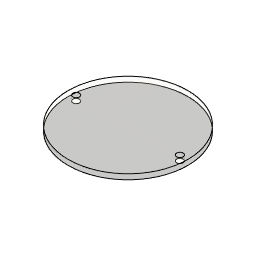
UNIT, SENSOR (L) (Autodesk Fusion 360 archive; units mm, degrees)
design "PLATE, COVER"
Autodesk Fusion 360 part; units mm, degrees
note: some values were not read from the file. Chosen so that the rebuilt part matches the saved one: which sketch regions a step uses.
sketch "Sketch1" plane through (0, 0, 0) normal (0, 1, 0) x (1, 0, 0)
  circle A0 centre (0, 0) radius 34.55
  dimension "d1" = 69.1
  constraint coincident A0.centre origin
  measures "d1" diameter of A0
extrude "Extrude1" add sketch "Sketch1" along normal blind 3
sketch "Sketch2" plane through (0, 3, 0) normal (0, 1, 0) x (-1, 0, 0)
  circle A0 centre (0, 0) radius 34.55
  line L0 (30, 0) -> (-30, 0) construction
  dimension "d4" = 60
  constraint horizontal L0
  constraint midpoint A0.centre L0
  measures "d4" distance of L0.start L0.end
hole "Hole1" at (-30, 3, 0) at (30, 3, 0) direction (0, -1, 0) diameter 3.8 end through all

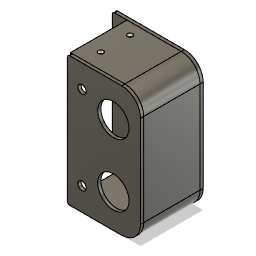
design "COVER, FIXTURE"
Autodesk Fusion 360 part; units mm, degrees
sketch "Sketch1" plane through (0, 0, 0) normal (0, 0, 1) x (1, 0, 0)
  line L0 (0, 31) -> (0, -31)
  line L1 (0, 31) -> (42, 31)
  line L2 (0, -31) -> (42, -31)
  line L3 (42, 31) -> (42, -31)
  dimension "d1" = 62
  dimension "d2" = 42
  constraint vertical L0
  constraint midpoint origin L0
  constraint perpendicular L0 L1
  constraint perpendicular L0 L2
  constraint perpendicular L1 L3
  measures "d1" distance of L0.start L0.end
  measures "d2" distance of L0.end L2.end
extrude "Extrude1" add sketch "Sketch1" along normal blind 1.5 makes body 1
fillet "Fillet3" radius 9 2 edges at (42, 31, 0.75) (42, -31, 0.75) on bodies 1
sketch "Sketch3" plane through (0, 0, 1.5) normal (0, 0, 1) x (1, 0, 0)
  arc A0 (33, -31) -> (42, -22) centre (33, -22) ccw
  line L0 (42, -22) -> (42, 22)
  arc A1 (42, 22) -> (33, 31) centre (33, 22) ccw
  line L1 (33, 31) -> (0, 31)
  line L2 (0, 31) -> (0, -31)
  line L3 (0, -31) -> (33, -31)
  line L4 (1.5, -29.5) -> (33, -29.5)
  arc A2 (33, -29.5) -> (40.5, -22) centre (33, -22) ccw
  line L5 (40.5, -22) -> (40.5, 22)
  arc A3 (40.5, 22) -> (33, 29.5) centre (33, 22) ccw
  line L6 (33, 29.5) -> (1.5, 29.5)
  line L7 (1.5, 29.5) -> (1.5, -29.5)
  line L8 (7, 31) -> (7, -31)
  dimension "d15" = -1.5
  dimension "d16" = 35
  constraint coincident L1 L8.start
  constraint coincident L3 L8.end
  constraint perpendicular L3 L8
  measures "d16" distance of L0 L8
extrude "Extrude3" add sketch "Sketch3" along normal blind 27 separate body contours A0 L0 A1 L1 L3 L4 A2 L5 A3 L6 L8 makes body 2
sketch "Sketch4" plane through (0, 0, 28.5) normal (0, 0, 1) x (1, 0, 0)
  line L0 (7, -29.5) -> (7, -31)
  line L1 (7, -31) -> (33, -31)
  arc A0 (33, -31) -> (42, -22) centre (33, -22) ccw
  line L2 (42, -22) -> (42, 22)
  arc A1 (42, 22) -> (33, 31) centre (33, 22) ccw
  line L3 (33, 31) -> (7, 31)
  line L4 (7, 31) -> (7, 29.5)
  line L5 (7, 29.5) -> (33, 29.5)
  arc A2 (40.5, 22) -> (33, 29.5) centre (33, 22) ccw
  line L6 (40.5, 22) -> (40.5, -22)
  arc A3 (33, -29.5) -> (40.5, -22) centre (33, -22) ccw
  line L7 (33, -29.5) -> (7, -29.5)
  line L8 (7, 31) -> (7, -31)
  constraint coincident L3.end L4.start
  constraint coincident L0.end L1.start
extrude "Extrude4" add sketch "Sketch4" along normal blind 1.5 separate body makes body 3
fillet "Fillet4" radius 1 4 edges at (0, 31, 0.75) (0, -31, 0.75) (7, -31, 29.25) (7, 31, 29.25) on bodies 1 3
sketch "Sketch5" plane through (0, 0, 30) normal (0, 0, 1) x (1, 0, 0)
  arc A0 (8, 31) -> (7, 30) centre (8, 30) ccw
  line L0 (7, 30) -> (7, -30)
  arc A1 (7, -30) -> (8, -31) centre (8, -30) ccw
  line L1 (8, -31) -> (33, -31)
  arc A2 (33, -31) -> (42, -22) centre (33, -22) ccw
  line L2 (42, -22) -> (42, 22)
  arc A3 (42, 22) -> (33, 31) centre (33, 22) ccw
  line L3 (33, 31) -> (8, 31)
  line L4 (29, 15) -> (29, -15) construction
  line L5 (0, 0) -> (29, 0) construction
  dimension "d23" = 30
  dimension "d24" = 22
  constraint perpendicular L1 L4
  constraint coincident L5.start origin
  constraint midpoint L4 L5.end
  constraint horizontal L5
  measures "d23" distance of L4.start L4.end
  measures "d24" distance of L0 L4
hole "Hole1" at (29, 15, 30) at (29, -15, 30) direction (0, 0, -1) diameter 15 depth 1.5 tip angle 180 bodies 3
sketch "Sketch6" plane through (0, 0, 30) normal (0, 0, 1) x (1, 0, 0)
  circle A0 centre (29, 15) radius 7.5
  circle A1 centre (29, -15) radius 7.5
  arc A2 (8, 31) -> (7, 30) centre (8, 30) ccw
  line L0 (7, 30) -> (7, -30)
  arc A3 (7, -30) -> (8, -31) centre (8, -30) ccw
  line L1 (8, -31) -> (33, -31)
  arc A4 (33, -31) -> (42, -22) centre (33, -22) ccw
  line L2 (42, -22) -> (42, 22)
  arc A5 (42, 22) -> (33, 31) centre (33, 22) ccw
  line L3 (33, 31) -> (8, 31)
  line L4 (14, 20) -> (14, -20) construction
  line L5 (0, 0) -> (14, 0) construction
  dimension "d28" = 40
  dimension "d29" = 7
  constraint vertical L4
  constraint coincident L5.start origin
  constraint midpoint L4 L5.end
  constraint horizontal L5
  measures "d28" distance of L4.start L4.end
  measures "d29" distance of L0 L4
hole "Hole2" at (14, 20, 30) at (14, -20, 30) direction (0, 0, -1) diameter 4 depth 1.5 tip angle 180 bodies 3
sketch "Sketch7" plane through (0, 31, 0) normal (0, 1, 0) x (-1, 0, 0)
  line L0 (-33, 1.5) -> (-7, 1.5)
  line L1 (-7, 1.5) -> (-7, 28.5)
  line L2 (-7, 28.5) -> (-33, 28.5)
  line L3 (-33, 28.5) -> (-33, 1.5)
  line L4 (-14, 7) -> (-14, 21) construction
  line L5 (-1, 0) -> (-33, 0) construction
  dimension "d33" = 7
  dimension "d34" = 14
  dimension "d35" = 7
  constraint vertical L4
  measures "d33" distance of L4.start L5
  measures "d34" distance of L4.start L4.end
  measures "d35" distance of L1 L4
hole "Hole3" at (14, 31, 7) at (14, 31, 21) direction (0, -1, 0) diameter 2.529 end through all bodies 2
thread "Thread1" "ISO Metric profile 3.0 M3x0.5 6H"
equation "d2 = 35 mm + 7 mm"
named bodies: "BACK", "SIDE", "FRONT"

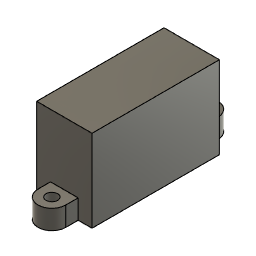
design "NAiS AMB 345908"
Autodesk Fusion 360 part; units mm, degrees
sketch "Sketch1" plane through (0, 0, 0) normal (0, 1, 0) x (1, 0, 0)
  line L0 (10, -23) -> (-10, -23)
  line L1 (-10, -23) -> (-10, 23)
  line L2 (-10, 23) -> (10, 23)
  line L3 (10, 23) -> (10, -23)
  line L4 (10, -23) -> (-10, 23) construction
  line L5 (-10, -23) -> (10, 23) construction
  dimension "d1" = 20
  dimension "d2" = 46
  constraint horizontal L0
  constraint perpendicular L0 L1
  constraint parallel L0 L2
  constraint parallel L1 L3
  constraint coincident L4 origin
  constraint coincident L5 origin
  measures "d1" distance of L0.start L0.end
  measures "d2" distance of L0.start L2.end
extrude "Extrude1" add sketch "Sketch1" along normal blind 29.7
sketch "Sketch2" plane through (0, 0, 0) normal (0, -1, 0) x (1, 0, 0)
  line L0 (-10, -23) -> (10, -23)
  line L1 (10, -23) -> (10, 23)
  line L2 (10, 23) -> (-10, 23)
  line L3 (-10, 23) -> (-10, -23)
  line L4 (5, -27.5) -> (5, 27.5)
  arc A0 (5, 27.5) -> (-5, 27.5) centre (0, 27.5) ccw
  line L5 (-5, 27.5) -> (-5, -27.5)
  arc A1 (-5, -27.5) -> (5, -27.5) centre (0, -27.5) ccw
  line L6 (0, -27.5) -> (0, 27.5) construction
  circle A2 centre (0, 27.5) radius 2.1
  circle A3 centre (0, -27.5) radius 2.1
  dimension "d5" = 55
  dimension "d6" = 10
  dimension "d7" = 4.2
  constraint tangent L4 A0
  constraint tangent A0 L5
  constraint parallel L4 L5
  constraint tangent L5 A1
  constraint tangent L4 A1
  constraint perpendicular L2 L6
  constraint midpoint L6 origin
  constraint concentric A0 A2
  constraint concentric A1 A3
  constraint equal A2 A3
  measures "d5" distance of A1.centre A0.centre
  measures "d6" distance of L4 L5
  measures "d7" diameter of A2
extrude "Extrude2" add sketch "Sketch2" against normal blind 7 contours L0 L4 L5 A1 | L2 L4 A0 L5

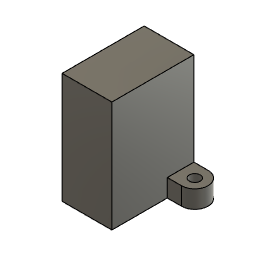
design "NAiS AMB 240903"
Autodesk Fusion 360 part; units mm, degrees
sketch "Sketch1" plane through (0, 0, 0) normal (0, 1, 0) x (1, 0, 0)
  line L0 (-7, -11.55) -> (7, -11.55)
  line L1 (7, -11.55) -> (7, 11.55)
  line L2 (7, 11.55) -> (-7, 11.55)
  line L3 (-7, 11.55) -> (-7, -11.55)
  line L4 (-7, -11.55) -> (7, 11.55) construction
  line L5 (7, -11.55) -> (-7, 11.55) construction
  dimension "d1" = 14
  dimension "d2" = 23.1
  constraint horizontal L0
  constraint perpendicular L0 L1
  constraint parallel L0 L2
  constraint parallel L1 L3
  constraint coincident L4 origin
  constraint coincident L5 origin
  measures "d1" distance of L1.end L2.end
  measures "d2" distance of L0.end L1.end
extrude "Extrude1" add sketch "Sketch1" along normal blind 31.2
sketch "Sketch2" plane through (0, 0, 0) normal (0, -1, 0) x (1, 0, 0)
  line L0 (-7, 11.55) -> (-7, -11.55)
  line L1 (-7, -11.55) -> (7, -11.55)
  line L2 (7, -11.55) -> (7, 11.55)
  line L3 (7, 11.55) -> (-7, 11.55)
  line L4 (-11, -11.55) -> (11, -11.55)
  arc A0 (11, -11.55) -> (11, -4.05) centre (11, -7.8) ccw
  line L5 (11, -4.05) -> (-11, -4.05)
  arc A1 (-11, -4.05) -> (-11, -11.55) centre (-11, -7.8) ccw
  line L6 (-11, -7.8) -> (11, -7.8) construction
  line L7 (-14.75, -7.8) -> (14.75, -7.8) construction
  circle A2 centre (-11, -7.8) radius 1.55
  circle A3 centre (11, -7.8) radius 1.55
  point P0 (0, -7.8)
  dimension "d5" = 22
  dimension "d6" = 29.5
  dimension "d7" = 3.1
  constraint tangent L4 A0
  constraint tangent A0 L5
  constraint parallel L4 L5
  constraint tangent L5 A1
  constraint tangent L4 A1
  constraint perpendicular L2 L6
  constraint midpoint L6 P0
  constraint vertical origin P0
  constraint coincident L1.end L4
  constraint midpoint A1 L7.start
  constraint midpoint A0 L7.end
  constraint concentric A1 A2
  constraint concentric A0 A3
  constraint equal A2 A3
  measures "d5" distance of A1.centre A0.centre
  measures "d6" distance of L7.start L7.end
  measures "d7" diameter of A3
extrude "Extrude2" add sketch "Sketch2" against normal blind 5 contours L0 L4 L5 A1 | L2 L4 A0 L5

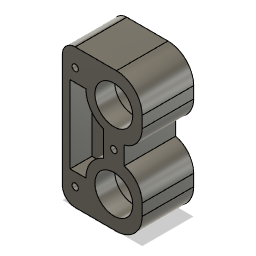
design "FIXTURE, LIGHT"
Autodesk Fusion 360 part; units mm, degrees
sketch "Sketch1" plane through (0, 0, 0) normal (0, 0, 1) x (1, 0, 0)
  line L0 (0, 27) -> (0, -27)
  line L1 (0, 27) -> (31, 27)
  line L2 (31, 27) -> (31, 12.5)
  arc A0 (24, 3.5) -> (31, 12.5) centre (21.7143, 12.5) ccw
  line L3 (24, 3.5) -> (24, -3.5)
  line L4 (0, 0) -> (24, 0) construction
  line L5 (0, -27) -> (31, -27)
  line L6 (31, -27) -> (31, -12.5)
  arc A1 (31, -12.5) -> (24, -3.5) centre (21.7143, -12.5) ccw
  dimension "d1" = 54
  dimension "d2" = 24
  dimension "d3" = 31
  dimension "d4" = 7
  dimension "d5" = 25
  constraint vertical L0
  constraint midpoint L4.start L0
  constraint perpendicular L0 L1
  constraint perpendicular L1 L2
  constraint tangent L2 A0
  constraint vertical L3
  constraint coincident L4.start origin
  constraint midpoint L3 L4.end
  constraint horizontal L4
  constraint perpendicular L0 L5
  constraint perpendicular L5 L6
  constraint tangent L6 A1
  constraint coincident L2 L6.end
  constraint equal A0 A1
  measures "d1" distance of L0.start L0.end
  measures "d2" distance of L0 L3
  measures "d3" distance of L0 L2
  measures "d4" distance of A0.start L3.end
  measures "d5" distance of L2.end L6.end
extrude "Extrude1" add sketch "Sketch1" along normal blind 20
fillet "Fillet1" radius 5 2 edges at (0, 27, 10) (0, -27, 10)
fillet "Fillet2" radius 10 2 edges at (31, 27, 10) (31, -27, 10)
sketch "Sketch2" plane through (0, 0, 20) normal (0, 0, 1) x (1, 0, 0)
  arc A0 (21, -27) -> (31, -17) centre (21, -17) ccw
  line L0 (31, -17) -> (31, -12.5)
  arc A1 (31, -12.5) -> (24, -3.5) centre (21.7143, -12.5) ccw
  line L1 (24, -3.5) -> (24, 3.5)
  arc A2 (24, 3.5) -> (31, 12.5) centre (21.7143, 12.5) ccw
  line L2 (31, 12.5) -> (31, 17)
  arc A3 (31, 17) -> (21, 27) centre (21, 17) ccw
  line L3 (21, 27) -> (5, 27)
  arc A4 (5, 27) -> (0, 22) centre (5, 22) ccw
  line L4 (0, 22) -> (0, -22)
  arc A5 (0, -22) -> (5, -27) centre (5, -22) ccw
  line L5 (5, -27) -> (21, -27)
  line L6 (20, 15) -> (20, -15) construction
  line L7 (0, 0) -> (20, 0) construction
  dimension "d12" = 30
  dimension "d13" = 20
  constraint vertical L6
  constraint coincident L7.start origin
  constraint midpoint L6 L7.end
  constraint horizontal L7
  measures "d12" distance of L6.start L6.end
  measures "d13" distance of L7.start L7.end
hole "Hole1" at (20, 15, 20) at (20, -15, 20) direction (0, 0, -1) diameter 14.7 end through all
sketch "Sketch3" plane through (0, 0, 0) normal (0, 0, -1) x (-1, 0, 0)
  circle A0 centre (-20, 15) radius 7.35
  circle A1 centre (-20, -15) radius 7.35
  arc A2 (-31, -17) -> (-21, -27) centre (-21, -17) ccw
  line L0 (-21, -27) -> (-5, -27)
  arc A3 (-5, -27) -> (0, -22) centre (-5, -22) ccw
  line L1 (0, -22) -> (0, 22)
  arc A4 (0, 22) -> (-5, 27) centre (-5, 22) ccw
  line L2 (-5, 27) -> (-21, 27)
  arc A5 (-21, 27) -> (-31, 17) centre (-21, 17) ccw
  line L3 (-31, 17) -> (-31, 12.5)
  arc A6 (-31, 12.5) -> (-24, 3.5) centre (-21.7143, 12.5) ccw
  line L4 (-24, 3.5) -> (-24, -3.5)
  arc A7 (-24, -3.5) -> (-31, -12.5) centre (-21.7143, -12.5) ccw
  line L5 (-31, -12.5) -> (-31, -17)
  line L6 (-20, 15) -> (-20, -15)
  constraint coincident A0.centre L6.start
  constraint coincident A1.centre L6.end
hole "Hole2" at (20, 15, 0) at (20, -15, 0) direction (0, 0, 1) diameter 16 depth 12.3 tip angle 180
sketch "Sketch4" plane through (0, 0, 20) normal (0, 0, 1) x (1, 0, 0)
  circle A0 centre (20, 15) radius 7.35
  circle A1 centre (20, -15) radius 7.35
  arc A2 (21, -27) -> (31, -17) centre (21, -17) ccw
  line L0 (31, -17) -> (31, -12.5)
  arc A3 (31, -12.5) -> (24, -3.5) centre (21.7143, -12.5) ccw
  line L1 (24, -3.5) -> (24, 3.5)
  arc A4 (24, 3.5) -> (31, 12.5) centre (21.7143, 12.5) ccw
  line L2 (31, 12.5) -> (31, 17)
  arc A5 (31, 17) -> (21, 27) centre (21, 17) ccw
  line L3 (21, 27) -> (5, 27)
  arc A6 (5, 27) -> (0, 22) centre (5, 22) ccw
  line L4 (0, 22) -> (0, -22)
  arc A7 (0, -22) -> (5, -27) centre (5, -22) ccw
  line L5 (5, -27) -> (21, -27)
  line L6 (3, 15) -> (3, -15)
  line L7 (3, -15) -> (9.15, -15)
  line L8 (3, 15) -> (9.15, 15)
  line L9 (16, 4.9142) -> (16, -4.9142)
  arc A8 (9.15, 15) -> (16, 4.9142) centre (20, 15) ccw
  arc A9 (16, -4.9142) -> (9.15, -15) centre (20, -15) ccw
  line L10 (0, 0) -> (3, 0) construction
  dimension "d20" = 3.5
  dimension "d21" = 8
  dimension "d22" = 3
  dimension "d23" = 30
  constraint vertical L6
  constraint perpendicular L6 L7
  constraint perpendicular L6 L8
  constraint vertical L9
  constraint coincident A0.centre A8.centre
  constraint coincident A1.centre A9.centre
  constraint coincident L7.end A9.end
  constraint coincident A8 L9.start
  constraint equal A8 A9
  constraint coincident L9.start A8.end
  constraint coincident L10.start origin
  constraint midpoint L6 L10.end
  constraint horizontal L10
  measures "d20" distance of A0 A8
  measures "d21" distance of L1 L9
  measures "d22" distance of L4 L6
  measures "d23" distance of L6.start L6.end
extrude "Extrude2" cut sketch "Sketch4" against normal blind 8.5 contours L6 L7 L8 L9 A8 A9
ref_plane "WorkPlane1" through (15.5, 0, 10) normal (0, 0, 1) x (1, 0, 0)
mirror "Mirror1" about plane through (15.5, 0, 10) normal (0, 0, 1) of "Extrude2"
sketch "Sketch5" plane through (0, 0, 20) normal (0, 0, 1) x (1, 0, 0)
  line L0 (9.15, -15) -> (3, -15)
  line L1 (3, -15) -> (3, 15)
  line L2 (3, 15) -> (9.15, 15)
  arc A0 (9.15, 15) -> (16, 4.9142) centre (20, 15) ccw
  line L3 (16, 4.9142) -> (16, -4.9142)
  arc A1 (16, -4.9142) -> (9.15, -15) centre (20, -15) ccw
  circle A2 centre (20, 15) radius 7.35
  circle A3 centre (20, -15) radius 7.35
  arc A4 (21, -27) -> (31, -17) centre (21, -17) ccw
  line L4 (31, -17) -> (31, -12.5)
  arc A5 (31, -12.5) -> (24, -3.5) centre (21.7143, -12.5) ccw
  line L5 (24, -3.5) -> (24, 3.5)
  arc A6 (24, 3.5) -> (31, 12.5) centre (21.7143, 12.5) ccw
  line L6 (31, 12.5) -> (31, 17)
  arc A7 (31, 17) -> (21, 27) centre (21, 17) ccw
  line L7 (21, 27) -> (5, 27)
  arc A8 (5, 27) -> (0, 22) centre (5, 22) ccw
  line L8 (0, 22) -> (0, -22)
  arc A9 (0, -22) -> (5, -27) centre (5, -22) ccw
  line L9 (5, -27) -> (21, -27)
  line L10 (5, 20) -> (5, -20) construction
  line L11 (5, 0) -> (20, 0) construction
  line L12 (20, 15) -> (20, -15) construction
  dimension "d28" = 5
  dimension "d29" = 40
  constraint perpendicular L2 L10
  constraint midpoint L10 L11.start
  constraint horizontal L11
  constraint horizontal origin L11.start
  constraint coincident A0.centre A2.centre
  constraint coincident A1.centre A3.centre
  constraint coincident L11.end L12
  measures "d28" distance of L8 L10
  measures "d29" distance of L10.start L10.end
hole "Hole3" at (5, 20, 20) at (20, 0, 20) at (5, -20, 20) direction (0, 0, -1) diameter 2.5 end through all

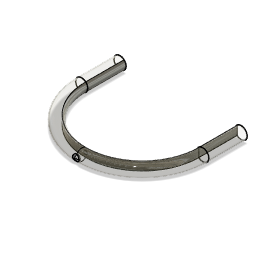
design "LIGHT, FIBER"
Autodesk Fusion 360 part; units mm, degrees
sketch "Sketch1" plane through (0, 0, 0) normal (1, 0, 0) x (0, 0, -1)
  circle A0 centre (0, 0) radius 6.5
  circle A1 centre (0, 0) radius 7.1
  dimension "d1" = 13
  dimension "d2" = 14.2
  constraint coincident A0.centre A1.centre
  constraint concentric A0 A1
  measures "d1" diameter of A0
  measures "d2" diameter of A1
sketch "Sketch2" plane through (0, 0, 0) normal (0, 1, 0) x (1, 0, 0)
  arc A0 (0, 0) -> (67.9, 67.9) centre (0, 67.9) ccw
  line L0 (67.9, 67.9) -> (67.9, 110.9)
  line L1 (0, -7.1) -> (0, 7.1) construction
  line L2 (60.8, 110.9) -> (75, 110.9) construction
  line L3 (0, 0) -> (-15, 0) construction
  line L4 (-67.9, 67.9) -> (-67.9, 110.9)
  arc A1 (-67.9, 67.9) -> (0, 0) centre (0, 67.9) ccw
  dimension "d3" = 118
  dimension "d4" = 14.2
  dimension "d5" = 75
  constraint coincident A0.start L3.start
  constraint tangent A0 L0
  constraint vertical L0
  constraint perpendicular L0 L2
  constraint midpoint L0.end L2
  constraint perpendicular L1 L3
  constraint tangent A0 L3
  constraint symmetric A0.start L1 L3.start
  constraint symmetric A0.end L1 L4.start
  constraint symmetric A0 L1 A1
  constraint symmetric L0.end L1 L4.end
  measures "d3" vertical distance of L0.end L1.start
  measures "d4" distance of L2.start L2.end
  measures "d5" distance of L1 L2.end
sweep "Sweep1" add profiles "Sketch1" path "Sketch2" along L4 A1 A0 L0 section 1 makes body 1
sketch "Sketch3" plane through (0, 0, -110.9) normal (0, 0, -1) x (-1, 0, 0)
  circle A0 centre (-67.9, 0) radius 6.5
  circle A1 centre (-67.9, 0) radius 7.1
  circle A2 centre (-67.9, 0) radius 6.5
  line L0 (-63.6, 4.8744) -> (-63.6, -4.8744)
  line L1 (-67.9, 0) -> (-61.4, 0) construction
  point P0 (-61.4, 0)
  dimension "d14" = 2.2
  constraint coincident A2 L0.start
  constraint coincident A2 L0.end
  constraint vertical L0
  constraint coincident A2 P0
  constraint coincident A0.centre A1.centre
  constraint coincident A0 P0
  constraint perpendicular L0 L1
  constraint coincident P0 L1.end
  measures "d14" distance of L0 P0
sweep "Sweep2" add profiles "Sketch3" path "Sketch2" along L4 A1 A0 L0 section 1 contours A0 A2 L0 picked at (-62.8882, 0.3052) separate body makes body 2
sweep "Sweep3" add profiles "Sketch3" path "Sketch2" along L4 A1 A0 L0 section 1 contours A0 A2 L0 picked at (-68.0098, 2.119) separate body makes body 3
ref_plane "WorkPlane1" through (0, 0, 7.1) normal (0, 0, 1) x (1, 0, 0)
sketch "Sketch4" plane through (0, 0, 7.1) normal (0, 0, 1) x (1, 0, 0)
hole "Hole1" at (0, 0, 7.1) direction (0, 0, -1) diameter 3.8 end through all counterbore diameter 7.1 counterbore depth 2 bodies 1 3
equation "d5 = ( 150 / 2 ) * 1 mm"
equation "d27 = ( 14.2 / 2 ) * 1 mm"
named bodies: "Pipe", "Resin"

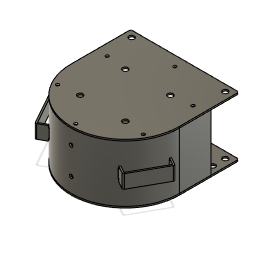
design "CABINET, SENSOR"
Autodesk Fusion 360 part; units mm, degrees
sketch "Sketch1" plane through (0, 0, 0) normal (0, 1, 0) x (1, 0, 0)
ref_plane "WorkPlane1" through (0, 33, 0) normal (0, 1, 0) x (0, 0, 1)
sketch "Sketch2" plane through (0, 33, 0) normal (0, 1, 0) x (1, 0, 0)
  circle A0 centre (0, 0) radius 60
  line L0 (-60, 0) -> (-60, 66)
  line L1 (-60, 66) -> (60, 66)
  line L2 (60, 66) -> (60, 0)
  point P0 (0, -60)
  dimension "d2" = 120
  dimension "d3" = 126
  constraint coincident A0.centre origin
  constraint coincident A0 L0.start
  constraint tangent A0 L0
  constraint vertical L0
  constraint perpendicular L0 L1
  constraint coincident A0 L2.end
  constraint tangent A0 L2
  constraint perpendicular L1 L2
  constraint coincident A0 P0
  constraint vertical A0.centre P0
  measures "d2" distance of L0.end L1.end
  measures "d3" distance of L1 P0
extrude "Extrude1" add sketch "Sketch2" against normal blind 1.6 makes body 1
sketch "Sketch3" plane through (0, 33, 0) normal (0, 1, 0) x (-1, 0, 0)
  arc A0 (60, 0) -> (-60, 0) centre (0, 0) ccw
  line L0 (-60, 0) -> (-60, -66)
  line L1 (-60, -66) -> (60, -66)
  line L2 (60, -66) -> (60, 0)
  circle A1 centre (0, 0) radius 55
  point P0 (0, 55)
  point P1 (-47.6314, 27.5)
  point P2 (-47.6314, -27.5)
  point P3 (0, -55)
  point P4 (47.6314, -27.5)
  point P5 (47.6314, 27.5)
  dimension "d6" = 110
  dimension "d8" = 360
  constraint coincident A0.centre A1.centre
  constraint coincident A1 P0
  constraint vertical A0.centre P0
  measures "d6" diameter of A1
hole "Hole1" at (0, 33, 55) at (-47.6314, 33, 27.5) at (-47.6314, 33, -27.5) at (0, 33, -55) at (47.6314, 33, -27.5) at (47.6314, 33, 27.5) direction (0, -1, 0) diameter 3.332 end through all bodies 1
thread "Thread1" "ISO Metric profile 4.0 M4x0.7 6H"
sketch "Sketch4" plane through (0, 33, 0) normal (0, 1, 0) x (-1, 0, 0)
  circle A0 centre (-47.6314, -27.5) radius 1.666
  circle A1 centre (47.6314, -27.5) radius 1.666
  circle A2 centre (0, 55) radius 1.666
  circle A3 centre (47.6314, 27.5) radius 1.666
  circle A4 centre (0, -55) radius 1.666
  circle A5 centre (-47.6314, 27.5) radius 1.666
  arc A6 (60, 0) -> (-60, 0) centre (0, 0) ccw
  line L0 (-60, 0) -> (-60, -66)
  line L1 (-60, -66) -> (60, -66)
  line L2 (60, -66) -> (60, 0)
  line L3 (52, -59) -> (-52, -59) construction
  line L4 (0, -66) -> (0, -59) construction
  dimension "d12" = 104
  dimension "d13" = 7
  constraint parallel L1 L3
  constraint midpoint L1 L4.start
  constraint midpoint L3 L4.end
  constraint vertical L4
  measures "d12" distance of L3.start L3.end
  measures "d13" distance of L1 L3
hole "Hole2" at (-52, 33, -59) at (52, 33, -59) direction (0, -1, 0) diameter 6 end through all bodies 1
fillet "Fillet1" radius 2 2 edges at (60, 32.2, -66) (-60, 32.2, -66) on bodies 1
mirror "Mirror1" about plane through (0, 0, 0) normal (0, 1, 0) of bodies 1 makes body 2
sketch "Sketch5" plane through (0, 33, 0) normal (0, 1, 0) x (-1, 0, 0)
  circle A0 centre (52, -59) radius 3
  circle A1 centre (-52, -59) radius 3
  circle A2 centre (-47.6314, -27.5) radius 1.666
  circle A3 centre (47.6314, -27.5) radius 1.666
  circle A4 centre (0, 55) radius 1.666
  circle A5 centre (47.6314, 27.5) radius 1.666
  circle A6 centre (0, -55) radius 1.666
  circle A7 centre (-47.6314, 27.5) radius 1.666
  arc A8 (58, -66) -> (60, -64) centre (58, -64) ccw
  line L0 (60, -64) -> (60, 0)
  arc A9 (60, 0) -> (-60, 0) centre (0, 0) ccw
  line L1 (-60, 0) -> (-60, -64)
  arc A10 (-60, -64) -> (-58, -66) centre (-58, -64) ccw
  line L2 (-58, -66) -> (58, -66)
  line L3 (-25, 25) -> (25, 25)
  line L4 (25, 25) -> (25, -25)
  line L5 (25, -25) -> (-25, -25)
  line L6 (-25, -25) -> (-25, 25)
  line L7 (-25, 25) -> (25, -25) construction
  line L8 (25, 25) -> (-25, -25) construction
  dimension "d21" = 50
  constraint horizontal L3
  constraint perpendicular L3 L4
  constraint parallel L3 L5
  constraint parallel L4 L6
  constraint coincident L7 A9.centre
  constraint coincident L8 A9.centre
  constraint coincident A9.centre origin
  constraint equal L5 L6
  measures "d21" distance of L3.start L5.end
hole "Hole3" at (-25, 33, -25) at (-25, 33, 25) at (25, 33, -25) at (25, 33, 25) direction (0, -1, 0) diameter 6 depth 1.6 tip angle 180 bodies 1
sketch "Sketch6" plane through (0, -33, 0) normal (0, -1, 0) x (1, 0, 0)
  circle A0 centre (-52, -59) radius 3
  circle A1 centre (52, -59) radius 3
  circle A2 centre (47.6314, -27.5) radius 1.666
  circle A3 centre (-47.6314, -27.5) radius 1.666
  circle A4 centre (0, 55) radius 1.666
  circle A5 centre (-47.6314, 27.5) radius 1.666
  circle A6 centre (0, -55) radius 1.666
  circle A7 centre (47.6314, 27.5) radius 1.666
  arc A8 (-60, -64) -> (-58, -66) centre (-58, -64) ccw
  line L0 (-58, -66) -> (58, -66)
  arc A9 (58, -66) -> (60, -64) centre (58, -64) ccw
  line L1 (60, -64) -> (60, 0)
  arc A10 (60, 0) -> (-60, 0) centre (0, 0) ccw
  line L2 (-60, 0) -> (-60, -64)
  circle A11 centre (0, 0) radius 40
  dimension "d25" = 80
  constraint concentric A10 A11
  measures "d25" diameter of A11
extrude "Extrude2" cut sketch "Sketch6" against normal up to surface (1.6 mm away) contours A11 bodies 2
sketch "Sketch7" plane through (0, -33, 0) normal (0, -1, 0) x (1, 0, 0)
  circle A0 centre (0, 0) radius 40
  circle A1 centre (-52, -59) radius 3
  circle A2 centre (52, -59) radius 3
  circle A3 centre (47.6314, -27.5) radius 1.666
  circle A4 centre (-47.6314, -27.5) radius 1.666
  circle A5 centre (0, 55) radius 1.666
  circle A6 centre (-47.6314, 27.5) radius 1.666
  circle A7 centre (0, -55) radius 1.666
  circle A8 centre (47.6314, 27.5) radius 1.666
  arc A9 (-60, -64) -> (-58, -66) centre (-58, -64) ccw
  line L0 (-58, -66) -> (58, -66)
  arc A10 (58, -66) -> (60, -64) centre (58, -64) ccw
  line L1 (60, -64) -> (60, 0)
  arc A11 (60, 0) -> (-60, 0) centre (0, 0) ccw
  line L2 (-60, 0) -> (-60, -64)
  line L3 (-52, -59) -> (52, -59)
  line L4 (52, -59) -> (52, -45)
  line L5 (52, -45) -> (-52, -45)
  line L6 (-52, -45) -> (-52, -59)
  dimension "d28" = 14
  constraint horizontal L3
  constraint vertical L4
  constraint horizontal L5
  constraint vertical L6
  constraint coincident A1.centre L3.start
  constraint coincident A2.centre L3.end
  measures "d28" distance of A1.centre L5.end
hole "Hole4" at (-52, -33, -45) at (52, -33, -45) direction (0, 1, 0) diameter 6 depth 1.6 tip angle 180 bodies 2
sketch "Sketch8" plane through (0, -33, 0) normal (0, -1, 0) x (1, 0, 0)
  circle A0 centre (-52, -45) radius 3
  circle A1 centre (52, -45) radius 3
  circle A2 centre (0, 0) radius 40
  circle A3 centre (-52, -59) radius 3
  circle A4 centre (52, -59) radius 3
  circle A5 centre (47.6314, -27.5) radius 1.666
  circle A6 centre (-47.6314, -27.5) radius 1.666
  circle A7 centre (0, 55) radius 1.666
  circle A8 centre (-47.6314, 27.5) radius 1.666
  circle A9 centre (0, -55) radius 1.666
  circle A10 centre (47.6314, 27.5) radius 1.666
  arc A11 (-60, -64) -> (-58, -66) centre (-58, -64) ccw
  line L0 (-58, -66) -> (58, -66)
  arc A12 (58, -66) -> (60, -64) centre (58, -64) ccw
  line L1 (60, -64) -> (60, 0)
  arc A13 (60, 0) -> (-60, 0) centre (0, 0) ccw
  line L2 (-60, 0) -> (-60, -64)
  line L3 (20, 42.5) -> (-20, 42.5)
  line L4 (-20, 42.5) -> (-20, -48.5)
  line L5 (-20, -48.5) -> (20, -48.5)
  line L6 (20, -48.5) -> (20, 42.5)
  line L7 (20, 42.5) -> (-20, -48.5) construction
  line L8 (-20, 42.5) -> (20, -48.5) construction
  point P0 (0, -3)
  dimension "d32" = 40
  dimension "d33" = 91
  dimension "d34" = 108.5
  constraint horizontal L3
  constraint perpendicular L3 L4
  constraint parallel L3 L5
  constraint parallel L4 L6
  constraint coincident L7 P0
  constraint coincident L8 P0
  constraint vertical A2.centre P0
  measures "d32" distance of L3.start L3.end
  measures "d33" distance of L3.start L5.end
  measures "d34" distance of L0 L3
hole "Hole5" at (-20, -33, 42.5) at (20, -33, 42.5) at (-20, -33, -48.5) at (20, -33, -48.5) direction (0, 1, 0) diameter 6 depth 1.6 tip angle 180 bodies 2
sketch "Sketch9" plane through (0, 31.4, 0) normal (0, -1, 0) x (1, 0, 0)
  circle A0 centre (25, -25) radius 3
  circle A1 centre (-25, -25) radius 3
  circle A2 centre (-25, 25) radius 3
  circle A3 centre (25, 25) radius 3
  arc A4 (-60, -64) -> (-58, -66) centre (-58, -64) ccw
  line L0 (-58, -66) -> (58, -66)
  arc A5 (58, -66) -> (60, -64) centre (58, -64) ccw
  line L1 (60, -64) -> (60, 0)
  arc A6 (60, 0) -> (-60, 0) centre (0, 0) ccw
  line L2 (-60, 0) -> (-60, -64)
  circle A7 centre (-52, -59) radius 3
  circle A8 centre (52, -59) radius 3
  circle A9 centre (47.6314, -27.5) radius 1.666
  circle A10 centre (-47.6314, -27.5) radius 1.666
  circle A11 centre (0, 55) radius 1.666
  circle A12 centre (-47.6314, 27.5) radius 1.666
  circle A13 centre (0, -55) radius 1.666
  circle A14 centre (47.6314, 27.5) radius 1.666
  arc A15 (-58.4, -64) -> (-58, -64.4) centre (-58, -64) ccw
  line L3 (-58, -64.4) -> (58, -64.4)
  arc A16 (58, -64.4) -> (58.4, -64) centre (58, -64) ccw
  line L4 (58.4, -64) -> (58.4, 0)
  arc A17 (58.4, 0) -> (-58.4, 0) centre (0, 0) ccw
  line L5 (-58.4, 0) -> (-58.4, -64)
  line L6 (-60, -35) -> (60, -35)
  dimension "d38" = -1.6
  dimension "d39" = 31
  constraint coincident L2 L6.start
  constraint coincident L1 L6.end
  constraint perpendicular L1 L6
  measures "d39" distance of L0 L6
extrude "Extrude3" add sketch "Sketch9" along normal up to surface (62.8 mm away) separate body contours L1 A6 L2 L4 A17 L5 L6 makes body 3
ref_plane "WorkPlane2" through (0, 7.1722, 60) normal (0, 0, 1) x (1, 0, 0)
sketch "Sketch10" plane through (0, 7.1722, 60) normal (0, 0, 1) x (1, 0, 0)
  line L0 (0, 7.8278) -> (0, -22.1722)
  line L1 (60, 24.2278) -> (60, -38.5722)
  line L2 (60, -7.1722) -> (0, -7.1722) construction
  dimension "d43" = 30
  constraint vertical L0
  constraint midpoint L1 L2.start
  constraint midpoint L0 L2.end
  constraint horizontal L2
  constraint coincident origin L0
  measures "d43" distance of L0.start L0.end
hole "Hole6" at (0, 15, 60) at (0, -15, 60) direction (0, 0, -1) diameter 4 depth 1.676 tip angle 180 bodies 3
ref_plane "WorkPlane3" through (0, 7.1722, 53.8) normal (0, 0, 1) x (1, 0, 0)
sketch "Sketch11" plane through (0, 7.1722, 53.8) normal (0, 0, 1) x (1, 0, 0)
  spline S0 degree 3 poles (2, 7.8278) (2, 8.0789) (1.9498, 8.3468) (1.7457, 8.8395) (1.5918, 9.0644) (1.2367, 9.4195) (1.0118, 9.5734) (0.519, 9.7776) (0.2511, 9.8278) (-0.2511, 9.8278) (-0.519, 9.7776) (-1.0118, 9.5734) (-1.2367, 9.4195) (-1.5918, 9.0644) (-1.7457, 8.8395) (-1.9498, 8.3468) (-2, 8.0789) (-2, 7.5766) (-1.9498, 7.3087) (-1.7457, 6.816) (-1.5918, 6.5911) (-1.2367, 6.236) (-1.0118, 6.0821) (-0.519, 5.878) (-0.2511, 5.8278) (0.2511, 5.8278) (0.519, 5.878) (1.0118, 6.0821) (1.2367, 6.236) (1.5918, 6.5911) (1.7457, 6.816) (1.9498, 7.3087) (2, 7.5766) (2, 7.8278) knots 0 0 0 0 0.075344 0.075344 0.150687 0.150687 0.226031 0.226031 0.301375 0.301375 0.376718 0.376718 0.452062 0.452062 0.527406 0.527406 0.602749 0.602749 0.678093 0.678093 0.753437 0.753437 0.82878 0.82878 0.904124 0.904124 0.979468 0.979468 1.054811 1.054811 1.130155 1.130155 1.205499 1.205499 1.205499 1.205499
  spline S1 degree 3 poles (2, -22.1722) (2, -21.9211) (1.9498, -21.6532) (1.7457, -21.1605) (1.5918, -20.9356) (1.2367, -20.5805) (1.0118, -20.4266) (0.519, -20.2224) (0.2511, -20.1722) (-0.2511, -20.1722) (-0.519, -20.2224) (-1.0118, -20.4266) (-1.2367, -20.5805) (-1.5918, -20.9356) (-1.7457, -21.1605) (-1.9498, -21.6532) (-2, -21.9211) (-2, -22.4234) (-1.9498, -22.6913) (-1.7457, -23.184) (-1.5918, -23.4089) (-1.2367, -23.764) (-1.0118, -23.9179) (-0.519, -24.122) (-0.2511, -24.1722) (0.2511, -24.1722) (0.519, -24.122) (1.0118, -23.9179) (1.2367, -23.764) (1.5918, -23.4089) (1.7457, -23.184) (1.9498, -22.6913) (2, -22.4234) (2, -22.1722) knots 0 0 0 0 0.075344 0.075344 0.150687 0.150687 0.226031 0.226031 0.301375 0.301375 0.376718 0.376718 0.452062 0.452062 0.527406 0.527406 0.602749 0.602749 0.678093 0.678093 0.753437 0.753437 0.82878 0.82878 0.904124 0.904124 0.979468 0.979468 1.054811 1.054811 1.130155 1.130155 1.205499 1.205499 1.205499 1.205499
  line L0 (-3.5, 9.8485) -> (-3.5, 5.807)
  line L1 (-3.5, 5.807) -> (0, 3.7863)
  line L2 (0, 3.7863) -> (3.5, 5.807)
  line L3 (3.5, 5.807) -> (3.5, 9.8485)
  line L4 (3.5, 9.8485) -> (0, 11.8692)
  line L5 (0, 11.8692) -> (-3.5, 9.8485)
  line L6 (-3.5, -20.1515) -> (-3.5, -24.193)
  line L7 (-3.5, -24.193) -> (0, -26.2137)
  line L8 (0, -26.2137) -> (3.5, -24.193)
  line L9 (3.5, -24.193) -> (3.5, -20.1515)
  line L10 (3.5, -20.1515) -> (0, -18.1308)
  line L11 (0, -18.1308) -> (-3.5, -20.1515)
  line L12 (0, 7.8278) -> (0, -22.1722) construction
  line L13 (-60, 24.2278) -> (-60, -38.5722) construction
  line L14 (0, -7.1722) -> (-60, -7.1722) construction
  point P0 (0, 7.8278)
  point P1 (0, -22.1722)
  dimension "d49" = 30
  dimension "d50" = 7
  constraint equal L5 L11
  constraint coincident P0 L12.start
  constraint vertical L12
  constraint coincident origin L12
  constraint coincident P1 L12.end
  constraint midpoint L12 L14.start
  constraint midpoint L13 L14.end
  constraint horizontal L14
  constraint vertical L3
  constraint coincident L3 L9.end
  measures "d49" distance of P0 P1
  measures "d50" distance of L6 L9
extrude "Extrude4" add sketch "Sketch11" along normal blind 4.567 separate body contours S0 | S1 | L0 L1 L2 L3 L4 L5 | L6 L7 L8 L9 L10 L11 makes body 4 at (-1.1667, 15.6736, 53.8) makes body 5 at (-1.1667, -14.3264, 53.8)
sketch "Sketch12" plane through (0, 0, 58.367) normal (0, 0, 1) x (1, 0, 0)
  line L0 (0, 19.0415) -> (-3.5, 17.0207)
  line L1 (-3.5, 17.0207) -> (-3.5, 12.9793)
  line L2 (-3.5, 12.9793) -> (0, 10.9585)
  line L3 (0, 10.9585) -> (3.5, 12.9793)
  line L4 (3.5, 12.9793) -> (3.5, 17.0207)
  line L5 (3.5, 17.0207) -> (0, 19.0415)
  line L6 (0, -10.9585) -> (-3.5, -12.9793)
  line L7 (-3.5, -12.9793) -> (-3.5, -17.0207)
  line L8 (-3.5, -17.0207) -> (0, -19.0415)
  line L9 (0, -19.0415) -> (3.5, -17.0207)
  line L10 (3.5, -17.0207) -> (3.5, -12.9793)
  line L11 (3.5, -12.9793) -> (0, -10.9585)
  line L12 (-3.5, -17.0207) -> (3.5, -12.9793) construction
  line L13 (0, 19.0415) -> (0, 10.9585) construction
  point P0 (0, 15)
  point P1 (0, -15)
  constraint coincident L7.end L8.start
  constraint coincident L10.end L11.start
  constraint coincident L0.start L5.end
  constraint coincident L2.end L3.start
  constraint midpoint P0 L13
  constraint midpoint P1 L12
hole "Hole7" at (0, 15, 58.367) at (0, -15, 58.367) direction (0, 0, -1) diameter 2.529 end through all bodies 4 5
thread "Thread2" "ISO Metric profile 3.0 M3x0.5 6H"
sketch "Sketch13" plane through (0, 0, 0) normal (0, 1, 0) x (1, 0, 0)
  arc A0 (-60, 0) -> (60, 0) centre (0, 0) ccw construction
  line L0 (60, 35) -> (60, 0) construction
  line L1 (0, 0) -> (59.4349, -8.2156) construction
  line L2 (0, 0) -> (38.2635, -46.2159) construction
  arc A1 (-58.4, 0) -> (58.4, 0) centre (0, 0) ccw construction
  line L3 (59.4349, -8.2156) -> (62.613, 14.7766) construction
  line L4 (38.2635, -46.2159) -> (56.7131, -30.9408) construction
  line L5 (-58, 66) -> (58, 66) construction
  point P0 (57.8499, -7.9965)
  point P1 (58.4, 35)
  dimension "d58" = 43.5
  dimension "d59" = 43
  dimension "d60" = 39.6
  dimension "d61" = 82.1
  constraint coincident A0.centre L1.start
  constraint coincident A0 L1.end
  constraint coincident A0 L2.end
  constraint coincident A1 P0
  constraint coincident L1 P0
  constraint tangent A0 L3
  constraint tangent A0 L4
  measures "d58" distance of L1.end L2.end
  measures "d59" distance of P0 P1
ref_plane "WorkPlane4" through (38.2454, -3.4982, 46.2308) normal (0.637424, 0, 0.770513) x (0.770513, 0, -0.637424)
ref_plane "WorkPlane5" through (59.4306, 17.418, 8.2467) normal (0.990509, 0, 0.137445) x (0.137445, 0, -0.990509)
sketch "Sketch14" plane through (38.2454, -3.4982, 46.2308) normal (0.637424, 0, 0.770513) x (0.770513, 0, -0.637424)
  line L0 (0.0234, 8.4982) -> (2.2234, 8.4982)
  line L1 (2.2234, 8.4982) -> (2.2234, -1.5018)
  line L2 (2.2234, -1.5018) -> (0.0234, -1.5018)
  line L3 (0.0234, -1.5018) -> (0.0234, 8.4982)
  point P0 (0.0234, 3.4982)
  dimension "d64" = 2.2
  dimension "d65" = 10
  constraint horizontal L0
  constraint vertical L1
  constraint horizontal L2
  constraint vertical L3
  constraint midpoint L3 P0
  measures "d64" distance of L0.start L0.end
  measures "d65" distance of L0.end L1.end
extrude "Extrude5" cut sketch "Sketch14" along normal up to surface end surface at (-9.3594, -4.9315, 57.6451) on bodies 3 bodies 3
sketch "Sketch15" plane through (59.4306, 17.418, 8.2467) normal (0.990509, 0, 0.137445) x (0.137445, 0, -0.990509)
  line L0 (0.0314, -12.418) -> (-2.1686, -12.418)
  line L1 (-2.1686, -12.418) -> (-2.1686, -22.418)
  line L2 (-2.1686, -22.418) -> (0.0314, -22.418)
  line L3 (0.0314, -22.418) -> (0.0314, -12.418)
  point P0 (0.0314, -17.418)
  dimension "d68" = 2.2
  dimension "d69" = 10
  constraint horizontal L0
  constraint vertical L1
  constraint horizontal L2
  constraint vertical L3
  constraint midpoint L3 P0
  measures "d68" distance of L0.start L0.end
  measures "d69" distance of L0.end L1.end
extrude "Extrude6" cut sketch "Sketch15" along normal up to surface end surface at (-9.3594, -4.9315, 57.6451) on bodies 3 bodies 3
mirror "Mirror2" about plane through (0, 0, 0) normal (1, 0, 0) of "Extrude5", "Extrude6"
sketch "Sketch16" plane through (0, 0, 0) normal (0, 1, 0) x (1, 0, 0)
  line L0 (39.014, -46.3478) -> (48.6233, -51.7015)
  line L1 (48.6233, -51.7015) -> (69.5513, -14.138)
  line L2 (69.5513, -14.138) -> (59.942, -8.7843)
  line L3 (59.4349, -8.2156) -> (38.2635, -46.2159) construction
  line L4 (39.8414, -44.8627) -> (47.9656, -49.389)
  line L5 (47.9656, -49.389) -> (67.2388, -14.7957)
  line L6 (67.2388, -14.7957) -> (59.1146, -10.2694)
  line L7 (39.014, -46.3478) -> (39.8414, -44.8627)
  line L8 (59.1146, -10.2694) -> (59.942, -8.7843)
  line L9 (48.8492, -27.2157) -> (57.6022, -32.0923) construction
  line L10 (59.0937, -10.3893) -> (57.5078, -10.1692) construction
  line L11 (39.9324, -44.7818) -> (38.9118, -43.5481) construction
  line L12 (39.9324, -44.7818) -> (59.0937, -10.3893) construction
  arc A0 (-60, 0) -> (60, 0) centre (0, 0) ccw construction
  point P0 (38.2635, -46.2159)
  point P1 (59.4349, -8.2156)
  dimension "d74" = 43
  dimension "d75" = 11
  dimension "d76" = -1.7
  constraint perpendicular L0 L1
  constraint perpendicular L1 L2
  constraint equal L0 L2
  constraint coincident P1 L3.start
  constraint coincident P0 L3.end
  constraint parallel L1 L3
  constraint perpendicular L2 L8
  constraint perpendicular L0 L7
  constraint midpoint L3 L9.start
  constraint midpoint L5 L9.end
  constraint perpendicular L3 L9
  constraint coincident L11.start L12.start
  constraint coincident L10.start L12.end
  constraint coincident L6.end A0
  measures "d74" distance of L0.end L1.end
  measures "d75" distance of L1.end L2.end
extrude "Extrude7" add sketch "Sketch16" along normal mid plane 15 separate body makes body 6
fillet "Fillet2" radius 1.5 2 edges at (69.5513, 0, 14.138) (48.6233, 0, 51.7015) on bodies 6
sketch "Sketch17" plane through (0, 7.5, 0) normal (0, 1, 0) x (-1, 0, 0)
  arc A0 (-47.3129, 50.9714) -> (-49.3533, 50.3911) centre (-48.0429, 49.6611) ccw
  line L0 (-49.3533, 50.3911) -> (-68.8212, 15.4483)
  arc A1 (-68.8212, 15.4483) -> (-68.2409, 13.4079) centre (-67.5109, 14.7183) ccw
  line L1 (-68.2409, 13.4079) -> (-59.942, 8.7843)
  line L2 (-59.942, 8.7843) -> (-59.1146, 10.2694)
  line L3 (-59.1146, 10.2694) -> (-67.2388, 14.7957)
  line L4 (-67.2388, 14.7957) -> (-47.9656, 49.389)
  line L5 (-47.9656, 49.389) -> (-39.8414, 44.8627)
  line L6 (-39.8414, 44.8627) -> (-39.014, 46.3478)
  line L7 (-39.014, 46.3478) -> (-47.3129, 50.9714)
  arc A2 (-66.992, 15.2387) -> (-66.7958, 14.5489) centre (-66.549, 14.9918) ccw
  arc A3 (-47.5226, 49.1422) -> (-48.2124, 48.946) centre (-47.7694, 48.6992) ccw
  dimension "d81" = 1
  dimension "d82" = 1
  constraint coincident L4 A2.start
  constraint coincident L3 A2.end
  constraint tangent L4 A2
  constraint tangent L3 A2
  constraint coincident L4 A3.end
  constraint coincident L5 A3.start
  constraint tangent L4 A3
  constraint tangent L5 A3
  measures "d81" distance of A1.centre A2.centre
  measures "d82" distance of A0.centre A3.centre
extrude "Extrude8" add sketch "Sketch17" against normal up to surface (15 mm away) contours L4 L5 A3 | L3 L4 A2 bodies 6
sketch "Sketch18" plane through (49.478, 0, 27.5661) normal (-0.87357, 0, -0.486699) x (-0.486699, 0, 0.87357)
  line L0 (-19.8, -7.5) -> (-19.8, 7.5)
  line L1 (-19.8, 7.5) -> (-21.5, 7.5)
  line L2 (-21.5, 7.5) -> (-21.5, -7.5)
  line L3 (-21.5, -7.5) -> (-19.8, -7.5)
  line L4 (-21.5, 5) -> (-19.8, 5)
  line L5 (-19.8, 5) -> (-19.8, -5)
  line L6 (-19.8, -5) -> (-21.5, -5)
  line L7 (-21.5, -5) -> (-21.5, 5)
  line L8 (21.5, -7.5) -> (21.5, 7.5)
  line L9 (21.5, 7.5) -> (19.8, 7.5)
  line L10 (19.8, 7.5) -> (19.8, -7.5)
  line L11 (19.8, -7.5) -> (21.5, -7.5)
  line L12 (21.5, 5) -> (19.8, 5)
  line L13 (19.8, 5) -> (19.8, -5)
  line L14 (19.8, -5) -> (21.5, -5)
  line L15 (21.5, -5) -> (21.5, 5)
  line L16 (19.8, 0) -> (21.5, 0) construction
  line L17 (-21.5, 0) -> (-19.8, 0) construction
  dimension "d85" = 10
  dimension "d86" = 10
  constraint horizontal L4
  constraint vertical L5
  constraint horizontal L6
  constraint vertical L7
  constraint coincident L0 L5.end
  constraint coincident L2 L4.start
  constraint horizontal L12
  constraint vertical L13
  constraint horizontal L14
  constraint vertical L15
  constraint coincident L10 L13.end
  constraint coincident L8 L12.start
  constraint midpoint L13 L16.start
  constraint midpoint L8 L16.end
  constraint horizontal L16
  constraint midpoint L2 L17.start
  constraint midpoint L5 L17.end
  constraint horizontal L17
  measures "d85" distance of L12 L14
  measures "d86" distance of L4 L6
extrude "Extrude9" add sketch "Sketch18" along normal blind 2 contours L0 L2 L4 L5 L6 L7 | L8 L10 L12 L13 L14 L15 bodies 6
mirror "Mirror3" about plane through (0, 0, 0) normal (1, 0, 0) of bodies 6 makes body 7
sketch "Sketch19" plane through (0, -33, 0) normal (0, -1, 0) x (1, 0, 0)
  circle A0 centre (-20, -48.5) radius 3
  circle A1 centre (-20, 42.5) radius 3
  circle A2 centre (20, 42.5) radius 3
  circle A3 centre (20, -48.5) radius 3
  circle A4 centre (-52, -45) radius 3
  circle A5 centre (52, -45) radius 3
  circle A6 centre (0, 0) radius 40
  circle A7 centre (-52, -59) radius 3
  circle A8 centre (52, -59) radius 3
  circle A9 centre (47.6314, -27.5) radius 1.666
  circle A10 centre (-47.6314, -27.5) radius 1.666
  circle A11 centre (0, 55) radius 1.666
  circle A12 centre (-47.6314, 27.5) radius 1.666
  circle A13 centre (0, -55) radius 1.666
  circle A14 centre (47.6314, 27.5) radius 1.666
  arc A15 (-60, -64) -> (-58, -66) centre (-58, -64) ccw
  line L0 (-58, -66) -> (58, -66)
  arc A16 (58, -66) -> (60, -64) centre (58, -64) ccw
  line L1 (60, -64) -> (60, 0)
  arc A17 (60, 0) -> (-60, 0) centre (0, 0) ccw
  line L2 (-60, 0) -> (-60, -64)
  line L3 (-43, 7) -> (43, 7) construction
  line L4 (0, 0) -> (0, 7) construction
  dimension "d91" = 86
  dimension "d92" = 73
  constraint horizontal L3
  constraint coincident A6.centre A17.centre
  constraint midpoint L3 L4.end
  constraint vertical L4
  measures "d91" distance of L3.start L3.end
  measures "d92" distance of L0 L3
hole "Hole8" at (-43, -33, 7) at (43, -33, 7) direction (0, 1, 0) diameter 3.332 depth 1.6 tip angle 180 bodies 2
thread "Thread3" "ISO Metric profile 4.0 M4x0.7 6H"
equation "d1 = ( 66 / 2 ) * 1 mm"
equation "d47 = -4.6 mm - 1.6 mm"
equation "d86 = d85"
named bodies: "TOP PLATE", "BOTTOM PLATE", "BODY", "TOP NUT", "BOTTOM NUT", "SPACER RIGHT", "SPACER LEFT"
